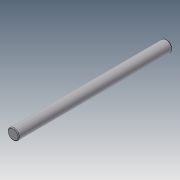
# Autodesk Inventor part: J008574
Saved by Autodesk Inventor 2018.3 (Build 223284000, 284)
## iProperties
Created: 2017-01-23
Material: ALUMINUM, 6061-T651
Vendor: HHMI: JRC - ID&F
Document SubType Name: Modeling
Designer: ARNOLDJ
Density: 2.7 g/cm^3
Appearance: Metal-AL-6061 (Machined)
Part Number: J008574
Description: NEUROPIXELS GEN 2 ADAPTER ROD
Project: COMMON
RuleStatus: InUse
AfterDocSave0: file://Part Number Cleaner
LAB/DEPT: APIG (SHARED RESOURCE)
REQUESTING SCIENTIST: COMMON
SURFACE ROUGHNESS: 32 Ra
DESIGN DEPARTMENT: HHMI: JRC - ID&F
SPECIAL FINISH: NONE
ALTERED ITEM PART NUMBER: N/A
ALTERED ITEM VENDOR: N/A
ALTERED ITEM DESCRIPTION: N/A
Author: ARNOLDJ
Revision Number: -
Autodesk Inventor part; units mm, degrees
ref_plane "YZ Plane" through (0, 0, 0) normal (1, 0, 0) x (0, 1, 0)
ref_plane "XZ Plane" through (0, 0, 0) normal (0, 1, 0) x (-1, 0, 0)
ref_plane "XY Plane" through (0, 0, 0) normal (0, 0, 1) x (1, 0, 0)
sketch "Sketch1" plane through (0, 0, 0) normal (0, 0, 1) x (1, 0, 0)
  circle A0 centre (0, 0) radius 3.175
  dimension "d0" = 6.35
  constraints: 1 centre point, 1 coincident
  measures "d0" diameter of A0
extrude "Extrusion1" add sketch "Sketch1" along normal blind 89.408
hole "Hole2" at (0, 0, 0) direction (0, 0, 1) diameter 4.0132 depth 29.21 tip angle 118 countersink diameter 4.5212 countersink angle 90
chamfer "Chamfer3" distance 0.381 angle 45 2 edges at (-3.175, 0, 89.408) (-3.175, 0, 0)
sketch "Sketch11" plane through (0, 0, 0) normal (1, 0, 0) x (0, 1, 0)
  line L0 (-2.0066, 29.21) -> (2.0066, 29.21) projected
  line L1 (0, 107.2896) -> (0, -17.8816) projected
  circle A0 centre (0, 28.448) radius 0.762 construction
  point P0 (0, 0)
  dimension "d65" = 1.524
  constraints: 1 centre point, 1 coincident, 1 point on line, 1 tangent
  measures "d65" diameter of A0
hole "Hole3" at (0, 0, 28.448) direction (-1, 0, 0) diameter 1.524 depth 3.81 tip angle 118
body "Solid1"
